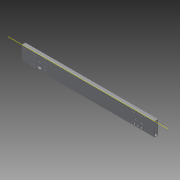
# Autodesk Inventor part: 4x1 boxbeam lengths
Saved by Autodesk Inventor 2015 (Build 190159000, 159)
## iProperties
Created: 2015-01-30
Part Number: 4x1 boxbeam lengths
Material: Generic
Document SubType Name: Modeling
Designer: chapale16
Density: 1 g/cm^3
Appearance: Default
Author: chapale16
Autodesk Inventor part; units mm, degrees
ref_plane "YZ Plane" through (0, 0, 0) normal (1, 0, 0) x (0, 1, 0)
ref_plane "XZ Plane" through (0, 0, 0) normal (0, 1, 0) x (-1, 0, 0)
ref_plane "XY Plane" through (0, 0, 0) normal (0, 0, 1) x (1, 0, 0)
sketch "Sketch1" plane through (0, 0, 0) normal (1, 0, 0) x (0, 1, 0)
  line L0 (0, 0) -> (-101.6, 0)
  line L1 (-101.6, 0) -> (-101.6, -25.4)
  line L2 (-101.6, -25.4) -> (0, -25.4)
  line L3 (0, -25.4) -> (0, 0)
  line L4 (-3.175, -3.175) -> (-98.425, -3.175)
  line L5 (-98.425, -3.175) -> (-98.425, -22.225)
  line L6 (-98.425, -22.225) -> (-3.175, -22.225)
  line L7 (-3.175, -22.225) -> (-3.175, -3.175)
  dimension "d0" = 101.6
  dimension "d1" = 25.4
  dimension "d2" = 3.175
  constraints: 16 end point, 4 parallel, 2 perpendicular, 1 horizontal, 3 other
  measures "d0" distance of L2.end L1.end
  measures "d1" distance of L1.end L0.end
  measures "d2" distance between parallel lines of L3 L7
extrude "Extrusion1" add sketch "Sketch1" along normal blind 965.2
sketch "Sketch2" plane through (0, -101.6, 0) normal (0, 0, 1) x (1, 0, 0)
  line L0 (909.1795, 114.4192) -> (797.5413, 105.3674)
  arc A0 (797.5413, 105.3674) -> (791.7045, 99.0382) centre (798.0545, 99.0382) ccw
  line L1 (791.7045, 99.0382) -> (791.7045, 2.8001)
  arc A1 (791.7045, 2.8001) -> (797.5413, -3.5291) centre (798.0545, 2.8001) ccw
  line L2 (797.5413, -3.5291) -> (909.1795, -12.5808)
  line L3 (909.1795, -12.5808) -> (910.8305, -12.5808)
  line L4 (910.8305, 114.4192) -> (910.8305, -12.5808)
  line L5 (910.8305, 114.4192) -> (909.1795, 114.4192)
  circle A2 centre (889.5947, 6.3422) radius 2.0447
  circle A3 centre (800.6947, 88.5112) radius 2.0447
  circle A4 centre (889.5947, 104.8942) radius 2.5527
  circle A5 centre (800.6947, 98.5442) radius 2.5527
  circle A6 centre (889.5947, 12.1842) radius 2.5527
  circle A7 centre (800.6947, 82.6692) radius 2.5527
  circle A8 centre (817.7127, 12.1842) radius 5.5562
  circle A9 centre (868.5127, 12.1842) radius 5.5562
  circle A10 centre (817.7127, 89.6542) radius 5.5562
  circle A11 centre (830.5665, 50.9192) radius 11.1061
  circle A12 centre (843.1127, 89.6542) radius 5.5562
  circle A13 centre (868.5127, 89.6542) radius 5.5562
  circle A14 centre (843.1127, 12.1842) radius 5.5562
  circle A15 centre (871.2827, 50.9192) radius 14.2811
  circle A16 centre (800.6947, 19.1692) radius 2.5527
  circle A17 centre (889.5947, 89.6542) radius 2.5527
  circle A18 centre (800.6947, 3.2942) radius 2.5527
  circle A19 centre (889.5947, -3.0558) radius 2.5527
  circle A20 centre (800.6947, 13.3272) radius 2.0447
  circle A21 centre (889.5947, 95.4962) radius 2.0447
  circle A22 centre (800.6947, 3.2942) radius 2.5527
  circle A23 centre (800.6947, 13.3272) radius 2.0447
  circle A24 centre (800.6947, 19.1692) radius 2.5527
  circle A25 centre (800.6947, 82.6692) radius 2.5527
  circle A26 centre (800.6947, 88.5112) radius 2.0447
  circle A27 centre (800.6947, 98.5442) radius 2.5527
  circle A28 centre (830.5665, 50.9192) radius 11.1061
  circle A29 centre (817.7127, 89.6542) radius 5.5563
  circle A30 centre (843.1127, 89.6542) radius 5.5562
  circle A31 centre (868.5127, 89.6542) radius 5.5562
  circle A32 centre (871.2827, 50.9192) radius 14.2811
  circle A33 centre (868.5127, 12.1842) radius 5.5562
  circle A34 centre (843.1127, 12.1842) radius 5.5562
  circle A35 centre (817.7127, 12.1842) radius 5.5562
  circle A36 centre (889.5947, 89.6542) radius 2.5527
  circle A37 centre (889.5947, 95.4962) radius 2.0447
  circle A38 centre (889.5947, 104.8942) radius 2.5527
  circle A39 centre (889.5947, 12.1842) radius 2.5527
  circle A40 centre (889.5947, 6.3422) radius 2.0447
  circle A41 centre (889.5947, -3.0558) radius 2.5527
  point P0 (0, 101.6)
  constraints: 42 centre point, 20 coincident, 20 concentric, 12 end point, 4 point on circle
extrude "Extrusion2" cut sketch "Sketch2" against normal blind 25.4 contours A2 | A3 | A4 | A5 | A6 | A7 | A8 | A9 | A10 | A11 | A12 | A13 | A14 | A15 | A16 | A17 | A18 | A19 | A20 | A21
sketch "Sketch3" plane through (0, -101.6, 0) normal (0, 0, 1) x (1, 0, 0)
  line L0 (190.5, -13.3248) -> (181.4483, 98.3133) projected
  arc A0 (181.4483, 98.3133) -> (175.119, 104.1502) centre (175.119, 97.8002) ccw projected
  line L1 (175.119, 104.1502) -> (78.881, 104.1502) projected
  arc A1 (78.881, 104.1502) -> (72.5517, 98.3133) centre (78.881, 97.8002) ccw projected
  line L2 (72.5517, 98.3133) -> (63.5, -13.3248) projected
  line L3 (63.5, -13.3248) -> (63.5, -14.9758) projected
  line L4 (190.5, -14.9758) -> (63.5, -14.9758) projected
  line L5 (190.5, -14.9758) -> (190.5, -13.3248) projected
  circle A2 centre (82.423, 6.2599) radius 2.0447 projected
  circle A3 centre (164.592, 95.1599) radius 2.0447 projected
  circle A4 centre (180.975, 6.2599) radius 2.5527 projected
  circle A5 centre (174.625, 95.1599) radius 2.5527 projected
  circle A6 centre (88.265, 6.2599) radius 2.5527 projected
  circle A7 centre (158.75, 95.1599) radius 2.5527 projected
  circle A8 centre (88.265, 78.1419) radius 5.5562 projected
  circle A9 centre (88.265, 27.3419) radius 5.5562 projected
  circle A10 centre (165.735, 78.1419) radius 5.5562 projected
  circle A11 centre (127, 65.2882) radius 11.1061 projected
  circle A12 centre (165.735, 52.7419) radius 5.5562 projected
  circle A13 centre (165.735, 27.3419) radius 5.5562 projected
  circle A14 centre (88.265, 52.7419) radius 5.5562 projected
  circle A15 centre (127, 24.572) radius 14.2811 projected
  circle A16 centre (95.25, 95.1599) radius 2.5527 projected
  circle A17 centre (165.735, 6.2599) radius 2.5527 projected
  circle A18 centre (79.375, 95.1599) radius 2.5527 projected
  circle A19 centre (73.025, 6.2599) radius 2.5527 projected
  circle A20 centre (89.408, 95.1599) radius 2.0447 projected
  circle A21 centre (171.577, 6.2599) radius 2.0447 projected
  circle A22 centre (79.375, 95.1599) radius 2.5527
  circle A23 centre (89.408, 95.1599) radius 2.0447
  circle A24 centre (95.25, 95.1599) radius 2.5527
  circle A25 centre (88.265, 78.1419) radius 5.5562
  circle A26 centre (127, 65.2882) radius 11.1061
  circle A27 centre (88.265, 52.7419) radius 5.5562
  circle A28 centre (88.265, 27.3419) radius 5.5562
  circle A29 centre (88.265, 6.2599) radius 2.5527
  circle A30 centre (82.423, 6.2599) radius 2.0447
  circle A31 centre (73.025, 6.2599) radius 2.5527
  circle A32 centre (127, 24.572) radius 14.2811
  circle A33 centre (165.735, 27.3419) radius 5.5562
  circle A34 centre (165.735, 6.2599) radius 2.5527
  circle A35 centre (171.577, 6.2599) radius 2.0447
  circle A36 centre (180.975, 6.2599) radius 2.5527
  circle A37 centre (165.735, 52.7419) radius 5.5563
  circle A38 centre (165.735, 78.1419) radius 5.5563
  circle A39 centre (164.592, 95.1599) radius 2.0447
  circle A40 centre (158.75, 95.1599) radius 2.5527
  circle A41 centre (174.625, 95.1599) radius 2.5527
  point P0 (0, 101.6)
  constraints: 20 centre point, 20 coincident, 20 concentric
extrude "Extrusion3" cut sketch "Sketch3" against normal blind 25.4 contours A2 | A3 | A4 | A5 | A6 | A7 | A8 | A9 | A10 | A11 | A12 | A13 | A14 | A15 | A16 | A17 | A18 | A19 | A20 | A21
body "Solid1"
